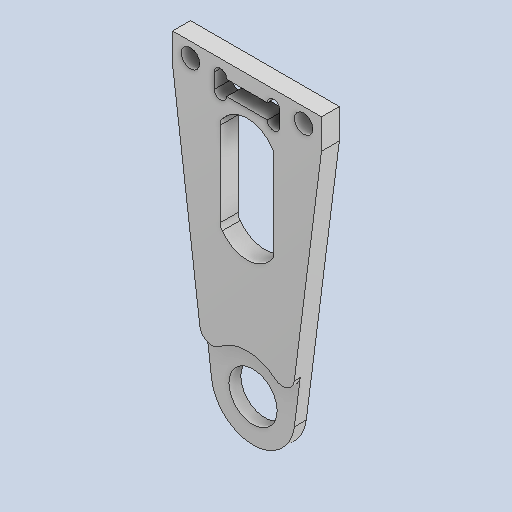
# Autodesk Inventor part: Leg_joint_slider_frame
Saved by Autodesk Inventor 2022.4 (Build 264492000, 492)
## iProperties
Created: 2021-10-17
Part Number: Leg_joint_slider_frame
Material: アルミニウム 2014-T4
Document SubType Name: Modeling
Designer: Masato Kubotera
Density: 2.8 g/cm^3
Appearance: 滑らか - 淡い灰色
Description: A2017 T3
Mass: 6.06844 g
Surface Area: 22.9593 cm^2
Volume: 2.1673 cm^3
Author: Masato Kubotera
Autodesk Inventor part; units mm, degrees
ref_plane "YZ Plane" through (0, 0, 0) normal (1, 0, 0) x (0, 1, 0)
ref_plane "XZ Plane" through (0, 0, 0) normal (0, 1, 0) x (-1, 0, 0)
ref_plane "XY Plane" through (0, 0, 0) normal (0, 0, 1) x (1, 0, 0)
derived "Leg_joint_roll_basis.ipt"
sketch "スケッチ1" plane through (0, 0, 0) normal (0, 0, 1) x (1, 0, 0)
  line L0 (0, 47.48) -> (0, -12.4) construction
  line L1 (-12.5, 47.48) -> (12.5, 47.48)
  line L2 (-12.5, 47.48) -> (-12.5, 42.48)
  line L3 (-12.5, 42.48) -> (-6.9432, -0.8896)
  arc A0 (-6.9432, -0.8896) -> (6.9432, -0.8896) centre (0, 0) ccw
  line L4 (-5.51, 45) -> (-3.41, 45) construction
  line L5 (5.51, 45) -> (5.51, 42.48)
  line L6 (5.51, 42.48) -> (3.41, 42.48) construction
  line L7 (-5.51, 42.48) -> (-5.51, 45)
  line L8 (-5.51, 45) -> (5.51, 42.48) construction
  line L9 (5.51, 45) -> (-5.51, 42.48) construction
  line L10 (-5.5, 44.99) -> (5.5, 44.99) construction
  line L11 (5.5, 44.99) -> (5.5, 42.49) construction
  line L12 (5.5, 42.49) -> (-5.5, 42.49) construction
  line L13 (-5.5, 42.49) -> (-5.5, 44.99) construction
  line L14 (-5.5, 44.99) -> (5.5, 42.49) construction
  line L15 (5.5, 44.99) -> (-5.5, 42.49) construction
  line L16 (-5.51, 43.74) -> (5.51, 43.74) construction
  arc A1 (-3.41, 45) -> (-5.51, 45) centre (-4.46, 45) ccw
  arc A2 (-5.51, 42.48) -> (-3.41, 42.48) centre (-4.46, 42.48) ccw
  circle A3 centre (-9.5, 45) radius 1.55
  line L17 (12.5, 42.48) -> (6.9432, -0.8896)
  line L18 (12.5, 47.48) -> (12.5, 42.48)
  circle A4 centre (9.5, 45) radius 1.55
  arc A5 (5.51, 45) -> (3.41, 45) centre (4.46, 45) ccw
  arc A6 (3.41, 42.48) -> (5.51, 42.48) centre (4.46, 42.48) ccw
  line L19 (-3.41, 45) -> (3.41, 45)
  line L20 (-3.41, 42.48) -> (-5.51, 42.48) construction
  line L21 (3.41, 42.48) -> (-3.41, 42.48)
  line L22 (3.41, 45) -> (5.51, 45) construction
  circle A7 centre (0, 0) radius 4.05
  line L23 (-13.5, 17) -> (13.5, 17) construction
  line L24 (13.5, 17) -> (13.5, -10) construction
  line L25 (13.5, -10) -> (-13.5, -10) construction
  line L26 (-13.5, -10) -> (-13.5, 17) construction
  line L27 (-13.5, 17) -> (13.5, -10) construction
  line L28 (13.5, 17) -> (-13.5, -10) construction
  arc A8 (-13.5, 18.35) -> (-13.5, 15.65) centre (-13.5, 17) ccw construction
  circle A9 centre (-13.5, -10) radius 1.35 construction
  line L29 (-24.81, 12.5) -> (-24.81, -5.5) construction
  circle A10 centre (-13.5, -10) radius 2.4 construction
  line L30 (-24.81, -5.5) -> (-14.2125, -12.4) construction
  line L31 (-21.75, 7.5) -> (-19.75, 7.5) construction
  line L32 (-19.75, 7.5) -> (-19.75, -0.5) construction
  line L33 (-19.75, -0.5) -> (-21.75, -0.5) construction
  line L34 (-21.75, -0.5) -> (-21.75, 7.5) construction
  line L35 (-21.75, 7.5) -> (-19.75, -0.5) construction
  line L36 (-19.75, 7.5) -> (-21.75, -0.5) construction
  line L37 (-21.76, 7.51) -> (-19.74, 7.51) construction
  line L38 (-19.74, 7.51) -> (-19.74, 5.41) construction
  line L39 (-19.74, -0.51) -> (-21.76, -0.51) construction
  line L40 (-21.76, -0.51) -> (-21.76, 1.59) construction
  line L41 (-21.76, 7.51) -> (-19.74, -0.51) construction
  line L42 (-19.74, 7.51) -> (-21.76, -0.51) construction
  arc A11 (-21.76, 7.51) -> (-21.76, 5.41) centre (-21.76, 6.46) ccw construction
  line L43 (-20.75, 7.51) -> (-20.75, -0.51) construction
  line L44 (-21.76, 3.5) -> (-19.74, 3.5) construction
  arc A12 (-19.74, 5.41) -> (-19.74, 7.51) centre (-19.74, 6.46) ccw construction
  arc A13 (-21.76, 1.59) -> (-21.76, -0.51) centre (-21.76, 0.54) ccw construction
  arc A14 (-19.74, -0.51) -> (-19.74, 1.59) centre (-19.74, 0.54) ccw construction
  line L45 (-24.81, 12.5) -> (-14.2125, 19.4) construction
  line L46 (-13.5, 18.35) -> (-13, 18.35) construction
  line L47 (-13.5, 15.65) -> (-13, 15.65) construction
  arc A15 (-13, 15.65) -> (-13, 18.35) centre (-13, 17) ccw construction
  line L48 (-21.76, 5.41) -> (-21.76, 7.51) construction
  line L49 (-21.76, 1.59) -> (-21.76, 5.41) construction
  line L50 (-19.74, 1.59) -> (-19.74, -0.51) construction
  line L51 (-19.74, 5.41) -> (-19.74, 1.59) construction
  line L52 (19.74, 5.41) -> (19.74, 1.59) construction
  line L53 (21.76, 1.59) -> (21.76, 5.41) construction
  arc A16 (21.76, 5.41) -> (21.76, 7.51) centre (21.76, 6.46) ccw construction
  line L54 (21.76, 7.51) -> (19.74, 7.51) construction
  arc A17 (19.74, 7.51) -> (19.74, 5.41) centre (19.74, 6.46) ccw construction
  arc A18 (21.76, -0.51) -> (21.76, 1.59) centre (21.76, 0.54) ccw construction
  line L55 (19.74, -0.51) -> (21.76, -0.51) construction
  arc A19 (19.74, 1.59) -> (19.74, -0.51) centre (19.74, 0.54) ccw construction
  line L56 (24.81, 12.5) -> (24.81, -5.5) construction
  line L57 (24.81, 12.5) -> (14.2125, 19.4) construction
  arc A20 (13, 18.35) -> (13, 15.65) centre (13, 17) ccw construction
  line L58 (13.5, 18.35) -> (13, 18.35) construction
  arc A21 (13.5, 15.65) -> (13.5, 18.35) centre (13.5, 17) ccw construction
  line L59 (24.81, -5.5) -> (14.2125, -12.4) construction
  circle A22 centre (13.5, -10) radius 1.35 construction
  line L60 (13.5, 15.65) -> (13, 15.65) construction
  line L61 (-14.2125, -12.4) -> (14.2125, -12.4) construction
  line L62 (-14.2125, 19.4) -> (-11.0486, 19.4) construction
  circle A23 centre (0, 18) radius 5.05 construction
  circle A24 centre (-13.5, 17) radius 2.4 construction
  arc A25 (-11.0486, 19.4) -> (11.0486, 19.4) centre (0, 18) ccw construction
  line L63 (11.0486, 19.4) -> (14.2125, 19.4) construction
  circle A26 centre (0, 26.5) radius 1.35 construction
  circle A27 centre (-8.5, 18) radius 1.35 construction
  circle A28 centre (0, 9.5) radius 1.35 construction
  circle A29 centre (8.5, 18) radius 1.35 construction
  arc A30 (-10.4884, 20.9672) -> (10.4884, 20.9672) centre (0, 18) ccw construction
  arc A31 (5.7734, 37.6333) -> (-5.7734, 37.6333) centre (0, 36) ccw construction
  line L64 (-5.7734, 37.6333) -> (-10.4884, 20.9672) construction
  line L65 (5.7734, 37.6333) -> (10.4884, 20.9672) construction
  circle A32 centre (0, 36) radius 2.25 construction
  circle A33 centre (0, 9.5) radius 2.4 construction
  circle A34 centre (0, 0) radius 2.25 construction
  circle A35 centre (0, 0) radius 1.55 construction
  line L66 (0, -3.187) -> (-0.9093, -2.662) construction
  line L67 (-2.76, -1.5935) -> (-2.76, -0.5435) construction
  line L68 (-2.76, 1.5935) -> (-1.8507, 2.1185) construction
  line L69 (0, 3.187) -> (2.76, 1.5935) construction
  line L70 (2.76, 1.5935) -> (2.76, 0.5435) construction
  line L71 (2.76, -1.5935) -> (1.8507, -2.1185) construction
  arc A36 (0.9093, 2.662) -> (-0.9093, 2.662) centre (0, 2.137) ccw construction
  arc A37 (-1.8507, 2.1185) -> (-2.76, 0.5435) centre (-1.8507, 1.0685) ccw construction
  arc A38 (-2.76, -0.5435) -> (-1.8507, -2.1185) centre (-1.8507, -1.0685) ccw construction
  arc A39 (-0.9093, -2.662) -> (0.9093, -2.662) centre (0, -2.137) ccw construction
  arc A40 (1.8507, -2.1185) -> (2.76, -0.5435) centre (1.8507, -1.0685) ccw construction
  arc A41 (2.76, 0.5435) -> (1.8507, 2.1185) centre (1.8507, 1.0685) ccw construction
  line L72 (-0.9093, 2.662) -> (0, 3.187) construction
  line L73 (-1.8507, 2.1185) -> (-0.9093, 2.662) construction
  line L74 (-2.76, 0.5435) -> (-2.76, 1.5935) construction
  line L75 (-2.76, -0.5435) -> (-2.76, 0.5435) construction
  line L76 (-1.8507, -2.1185) -> (-2.76, -1.5935) construction
  line L77 (-0.9093, -2.662) -> (-1.8507, -2.1185) construction
  line L78 (0.9093, -2.662) -> (0, -3.187) construction
  line L79 (1.8507, -2.1185) -> (0.9093, -2.662) construction
  line L80 (2.76, -0.5435) -> (2.76, -1.5935) construction
  line L81 (2.76, 0.5435) -> (2.76, -0.5435) construction
  circle A42 centre (0, 0) radius 3 construction
  arc A43 (4.45, 38.3875) -> (-4.45, 38.3875) centre (0, 36) ccw
  line L82 (-4.45, 38.3875) -> (-4.45, 23.0684)
  arc A44 (-4.45, 23.0684) -> (4.45, 23.0684) centre (0, 25.4558) ccw
  line L83 (4.45, 38.3875) -> (4.45, 23.0684)
  arc A45 (7.1574, 0.782) -> (-7.1574, 0.782) centre (0, 0) ccw
  circle A46 centre (0, 0) radius 36 construction
  line L84 (-18, 18) -> (-25.4558, 25.4558) construction
  circle A47 centre (0, 18) radius 18 construction
  arc A48 (-4.1532, 38.8729) -> (-4.45, 37.8184) centre (-3.4393, 38.103) ccw
  line L85 (-4.45, 30.7279) -> (4.45, 30.7279) construction
  arc A49 (4.45, 37.8184) -> (4.1532, 38.8729) centre (3.4393, 38.103) ccw
  arc A50 (-4.45, 23.6374) -> (-4.1532, 22.5829) centre (-3.4393, 23.3529) ccw
  arc A51 (4.1532, 22.5829) -> (4.45, 23.6374) centre (3.4393, 23.3529) ccw
  point P0 (0, 43.74)
  point P1 (0, 3.5)
  point P2 (-20.75, 3.5)
  point P3 (-24.81, 3.5)
  point P4 (-13.5, 3.5)
  point P5 (4.1532, 22.5829)
  point P6 (-4.1532, 22.5829)
  point P7 (-4.45, 23.6374)
  point P8 (4.1532, 38.8729)
  point P9 (4.45, 37.8184)
  point P10 (4.45, 23.6374)
  dimension "d1" = 8.9
  dimension "d2" = 5.05
  dimension "d3" = 5.05
  dimension "d8" = 7.2
  dimension "d11" = 45
  dimension "d12" = 10.5442
  dimension "d13" = 72
  dimension "d15" = 10.5442
  dimension "d16" = 1.05
  measures "d1" distance between parallel lines of L82 L83
  measures "d2" radius of A43
  measures "d3" radius of A44
  measures "d8" radius of A45
  measures "d11" angle to the sketch x axis of L84
  measures "d12" distance of L84.start L84.end
  measures "d13" diameter of A46
  measures "d15" distance of A43.centre A44.centre
  measures "d16" radius of A48
extrude "押し出し1" add sketch "スケッチ1" along normal blind 3 contours L1 L18 L17 A45 L3 L2
extrude "押し出し2" add sketch "スケッチ1" along normal blind 2 contours A45 L17 A0 L3
fillet "フィレット1" radius 2 2 edges at (-7.1574, 0.782, 2.5) (7.1574, 0.782, 2.5)
equation "\"d3\" = d2"
equation "\"d15\" = d12"
